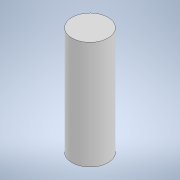
# Autodesk Inventor part: azimuthPost
Saved by Autodesk Inventor 2021 (Build 250183000, 183)
## iProperties
Created: 2020-07-19
Part Number: azimuthPost
Material: Generic
Document SubType Name: Modeling
Designer: robst
Density: 1 g/cm^3
Appearance: Default
Author: robst
Autodesk Inventor part; units mm, degrees
ref_plane "YZ Plane" through (0, 0, 0) normal (1, 0, 0) x (0, 1, 0)
ref_plane "XZ Plane" through (0, 0, 0) normal (0, 1, 0) x (-1, 0, 0)
ref_plane "XY Plane" through (0, 0, 0) normal (0, 0, 1) x (1, 0, 0)
sketch "Sketch1" plane through (0, 0, 0) normal (0, 1, 0) x (-1, 0, 0)
  circle A0 centre (0, 0) radius 12.7
  dimension "d0" = 25.4
  constraints: 1 centre point, 1 coincident
  measures "d0" diameter of A0
extrude "Extrusion1" add sketch "Sketch1" along normal mid plane 76.2
body "Solid1"
